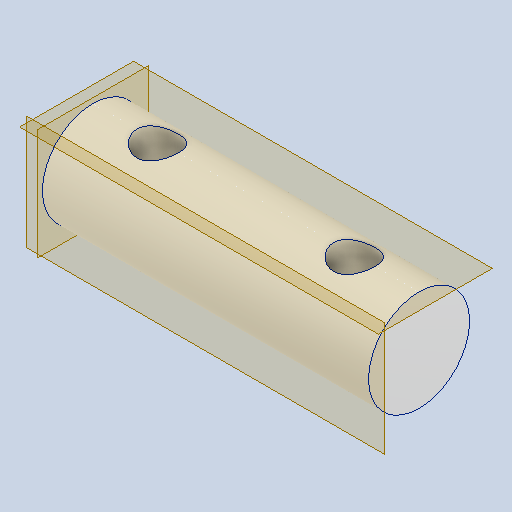
# Autodesk Inventor part: part2
Saved by Autodesk Inventor 2025.2 (Build 292293000, 293)
## iProperties
Created: 2025-02-28
Part Number: part2
Material: アルミニウム 6061
Document SubType Name: Modeling
Designer: haruy
Density: 2.7 g/cm^3
Appearance: アルミニウム - フラット
Author: haruy
Autodesk Inventor part; units mm, degrees
sketch "スケッチ1" plane through (0, 0, 0) normal (1, 0, 0) x (0, 1, 0)
  circle A0 centre (0, 0) radius 3.9
  dimension "d0" = 7.8
  constraints: 1 centre point, 1 coincident
  measures "d0" diameter of A0
extrude "押し出し1" add sketch "スケッチ1" along normal blind 25.2
ref_plane "作業平面1" through (0, 3.9, 0) normal (0, 1, 0) x (-1, 0, 0)
sketch "スケッチ2" plane through (0, 3.9, 0) normal (0, 1, 0) x (-1, 0, 0)
  line L0 (0, 3.9) -> (0, -3.9) projected
  line L1 (-25.2, 3.9) -> (-25.2, -3.9) projected
  point P0 (0, 0)
  point P1 (-5, 0)
  point P2 (-20.2, 0)
  dimension "d3" = 5
  dimension "d4" = 5
  measures "d3" distance from line of point (-5, 0) L0
  measures "d4" distance from line of L1 point (-20.2, 0)
hole "穴1" at (5, 3.9, 0) at (20.2, 3.9, 0) direction (0, -1, 0) diameter 3.2 end through all
ref_plane "作業平面2" through (0, 0, 3.9) normal (0, 0, 1) x (1, 0, 0)
